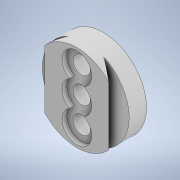
# Autodesk Inventor part: hockey puck
Saved by Autodesk Inventor 2020 (Build 240168000, 168)
## iProperties
Created: 2020-02-19
Part Number: hockey puck
Material: Generic
Document SubType Name: Modeling
Designer: Ball
Density: 1 g/cm^3
Appearance: Default
Author: Ball
Autodesk Inventor part; units mm, degrees
ref_plane "YZ Plane" through (0, 0, 0) normal (1, 0, 0) x (0, 1, 0)
ref_plane "XZ Plane" through (0, 0, 0) normal (0, 1, 0) x (-1, 0, 0)
ref_plane "XY Plane" through (0, 0, 0) normal (0, 0, 1) x (1, 0, 0)
sketch "Sketch1" plane through (0, 0, 0) normal (0, 0, 1) x (1, 0, 0)
  circle A0 centre (0, 0) radius 15.875
  dimension "d0" = 31.75
  constraints: 1 centre point, 1 coincident
  measures "d0" diameter of A0
extrude "Extrusion1" add sketch "Sketch1" along normal blind 6.35
sketch "Sketch2" plane through (0, 0, 0) normal (0, 1, 0) x (-1, 0, 0)
  line L0 (15.875, 6.35) -> (-15.875, 6.35) projected
  line L1 (0, 6.35) -> (-6.604, 6.35)
  line L2 (0, 6.35) -> (6.604, 6.35)
  line L3 (0, 9.6012) -> (-11.684, 9.6012)
  line L4 (0, 9.6012) -> (11.684, 9.6012)
  line L5 (11.684, 9.6012) -> (6.604, 6.35)
  line L6 (-6.604, 6.35) -> (-11.684, 9.6012)
  line L7 (0, 6.35) -> (0, 9.6012)
  point P0 (0, 0)
  dimension "d8" = 13.208
  dimension "d9" = 3.2512
  dimension "d10" = 23.368
  dimension "d29" = 11.684
  dimension "d30" = 6.604
  constraints: 14 end point, 2 point on line, 1 horizontal, 1 midpoint, 1 perpendicular
  measures "d8" distance of L1.end L2.end
  measures "d9" distance between parallel lines of L0 L3
  measures "d10" distance of L3.end L4.end
  measures "d29" distance of L3.start L3.end
  measures "d30" distance from line of L1.end L7
extrude "Extrusion2" add sketch "Sketch2" along normal mid plane 31.75
sketch "Sketch3" plane through (-11.684, 15.875, 9.6012) normal (0, 0, 1) x (1, 0, 0)
  circle A0 centre (11.684, -15.875) radius 15.875
  line L0 (0, -31.75) -> (0, 0) projected
  circle A1 centre (11.684, -15.875) radius 19.7112
  constraints: 2 coincident, 1 centre point, 3 other
extrude "Extrusion3" cut sketch "Sketch3" against normal blind 3.2512 contours A0 L0 A1 | A0 L0 A1
sketch "Sketch4" plane through (0, 0, 6.35) normal (0, 0, 1) x (1, 0, 0)
  circle A0 centre (0, 0) radius 3.1623
  circle A1 centre (0, 9.4742) radius 3.1623
  circle A2 centre (0, -9.4742) radius 3.1623
  dimension "d15" = 6.3246
  dimension "d16" = 6.3246
  dimension "d17" = 6.3246
  dimension "d18" = 9.4742
  dimension "d19" = 9.4742
  constraints: 3 centre point, 1 coincident
  measures "d15" diameter of A0
  measures "d16" diameter of A1
  measures "d17" diameter of A2
  measures "d18" distance of point (0, 0) A2.centre
  measures "d19" distance of point (0, 0) A1.centre
extrude "Extrusion4" cut sketch "Sketch4" along normal through all both and the other way through all
sketch "Sketch5" plane through (0, 0, 9.6012) normal (0, 0, 1) x (1, 0, 0)
  circle A0 centre (0, 9.4742) radius 3.1623 projected
  arc A1 (2.6656, 4.7371) -> (-2.6656, 4.7371) centre (0, 9.4742) ccw
  circle A2 centre (0, -9.4742) radius 3.1623 projected
  arc A3 (-2.6656, -4.7371) -> (2.6656, -4.7371) centre (0, -9.4742) ccw
  arc A4 (-2.6656, 4.7371) -> (-2.6656, -4.7371) centre (0, 0) ccw
  arc A5 (2.6656, -4.7371) -> (2.6656, 4.7371) centre (0, 0) ccw
  dimension "d23" = 10.8712
  dimension "d24" = 10.8712
  constraints: 8 point on circle, 4 centre point, 2 coincident
  measures "d23" diameter of A1
  measures "d24" diameter of A3
extrude "Extrusion5" cut sketch "Sketch5" against normal blind 1.778
body "Solid1"
